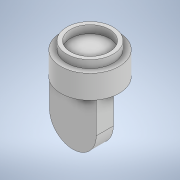
# Autodesk Inventor part: Shoulder1
Saved by Autodesk Inventor 2022 (Build 260153000, 153)
## iProperties
Created: 2021-10-29
Part Number: Shoulder1
Material: Generic
Document SubType Name: Modeling
Designer: Mark Maara
Density: 1 g/cm^3
Appearance: Default
Author: Mark Maara
Autodesk Inventor part; units mm, degrees
ref_plane "YZ Plane" through (0, 0, 0) normal (1, 0, 0) x (0, 1, 0)
ref_plane "XZ Plane" through (0, 0, 0) normal (0, 1, 0) x (-1, 0, 0)
ref_plane "XY Plane" through (0, 0, 0) normal (0, 0, 1) x (1, 0, 0)
sketch "Sketch1" plane through (0, 0, 0) normal (0, 1, 0) x (-1, 0, 0)
  circle A0 centre (0, 0) radius 37.5
  dimension "d0" = 75
  constraints: 1 centre point, 1 coincident
  measures "d0" diameter of A0
extrude "Extrusion1" add sketch "Sketch1" along normal blind 30
sketch "Sketch6" plane through (0, 30, 0) normal (0, 1, 0) x (1, 0, 0)
  circle A0 centre (0, 0) radius 30
  circle A1 centre (0, 0) radius 25
  circle A2 centre (0, 0) radius 7.5
  dimension "d16" = 60
  dimension "d17" = 50
  dimension "d28" = 15
  constraints: 3 centre point, 3 coincident
  measures "d16" diameter of A0
  measures "d17" diameter of A1
  measures "d28" diameter of A2
extrude "Extrusion5" add sketch "Sketch6" along normal blind 10 contours A0
sketch "Sketch9" plane through (0, 0, 0) normal (0, 0, 1) x (1, 0, 0)
  line L0 (0, 0) -> (30, 0)
  line L1 (30, 0) -> (30, -40)
  line L2 (30, -40) -> (0, -40)
  line L3 (0, -40) -> (0, 0)
  circle A0 centre (0, -40) radius 30
  line L4 (-30, 0) -> (-30, -40)
  line L5 (0, 0) -> (-30, 0)
  line L6 (37.5, 30) -> (-37.5, 30) projected
  point P0 (-30, -40)
  point P1 (30, -40)
  dimension "d38" = 40
  dimension "d40" = 60
  dimension "d41" = 30
  dimension "d44" = 0
  constraints: 12 end point, 3 parallel, 2 symmetric about line, 1 centre point, 1 horizontal, 1 perpendicular
  measures "d38" distance of L0.end L1.end
  measures "d40" diameter of A0
  measures "d41" distance of L1.end L2.end
  measures "d44" distance of L2.end A0.centre
extrude "Extrusion8" add sketch "Sketch9" along normal blind 22
body "Solid1"
